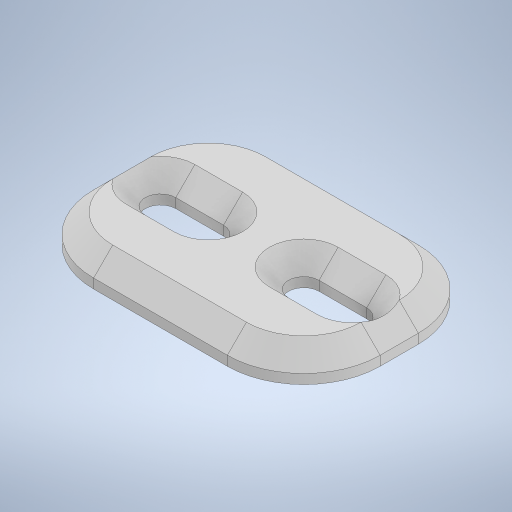
# Autodesk Inventor part: synth-straight-bracket
Saved by Autodesk Inventor 2024.1 (Build 281209000, 209)
## iProperties
Created: 2025-02-09
Part Number: synth-straight-bracket
Material: Generic
Document SubType Name: Modeling
Designer: iwheard
Density: 1 g/cm^3
Appearance: Default
Author: iwheard
Autodesk Inventor part; units mm, degrees
ref_plane "YZ Plane" through (0, 0, 0) normal (1, 0, 0) x (0, 1, 0)
ref_plane "XZ Plane" through (0, 0, 0) normal (0, 1, 0) x (-1, 0, 0)
ref_plane "XY Plane" through (0, 0, 0) normal (0, 0, 1) x (1, 0, 0)
sketch "Sketch1" plane through (0, 0, 0) normal (0, 1, 0) x (-1, 0, 0)
  line L0 (0, -20) -> (-30, -20)
  line L1 (-30, -20) -> (-30, 0)
  line L2 (-30, 0) -> (0, 0)
  line L3 (0, 0) -> (0, -20)
  dimension "d0" = 20
  dimension "d1" = 30
  constraints: 8 end point, 2 parallel, 1 coincident, 1 horizontal, 1 perpendicular
  measures "d0" distance between parallel lines of L2 L0
  measures "d1" distance between parallel lines of L3 L1
extrude "Extrusion1" add sketch "Sketch1" along normal blind 3
sketch "Sketch10" plane through (0, 3, 0) normal (0, 1, 0) x (1, 0, 0)
  circle A0 centre (5, 10) radius 1.6
  circle A1 centre (25, 10) radius 1.6
  line L0 (30, 20) -> (0, 20) projected
  line L1 (0, 0) -> (30, 0) projected
  line L2 (0, 20) -> (0, 0) projected
  line L3 (30, 0) -> (30, 20) projected
  line L4 (5, 10) -> (10, 10) construction
  line L5 (5, 8.4) -> (10, 8.4)
  line L6 (10, 11.6) -> (5, 11.6)
  arc A2 (5, 11.6) -> (5, 8.4) centre (5, 10) ccw
  arc A3 (10, 8.4) -> (10, 11.6) centre (10, 10) ccw
  line L7 (25, 10) -> (20, 10) construction
  line L8 (25, 8.4) -> (20, 8.4)
  line L9 (20, 11.6) -> (25, 11.6)
  arc A4 (25, 8.4) -> (25, 11.6) centre (25, 10) ccw
  arc A5 (20, 11.6) -> (20, 8.4) centre (20, 10) ccw
  point P0 (7.5, 10)
  point P1 (22.5, 10)
  dimension "d66" = 3.2
  dimension "d64" = 20
  dimension "d65" = 10
  dimension "d67" = 5
  dimension "d68" = 20
  dimension "d69" = 5
  dimension "d79" = 5
  dimension "d80" = 5
  constraints: 16 end point, 8 point on circle, 8 tangent, 4 centre point, 2 midpoint, 2 parallel, 1 horizontal, 1 horizontal alignment, 1 point on line, 6 other
  measures "d64" distance between parallel lines of L0 L1
  measures "d65" distance from line of L1 L4.start
  measures "d67" distance from line of L2 L4.start
  measures "d68" distance of L7.start L4.start
  measures "d69" distance from line of L3 L7.start
  measures "d79" distance of L4.end L4.start
  measures "d80" distance of L7.start L7.end
extrude "Extrusion6" cut sketch "Sketch10" against normal through all contours A0 | A0 L6 A3 L5 | A1 | A1 L8 A5 L9
fillet "Fillet5" radius 8 4 edges at (0, 1.5, 0) (0, 1.5, -20) (30, 1.5, -20) (30, 1.5, 0)
chamfer "Chamfer5" distance 2 angle 45 2 edges at (3.4, 3, -10) (26.6, 3, -10)
chamfer "Chamfer6" distance 2 angle 45 8 edges at (15, 3, 0) (27.6569, 3, -2.3431) (30, 3, -10) (27.6569, 3, -17.6569) (15, 3, -20) (2.3431, 3, -17.6569) (0, 3, -10) (2.3431, 3, -2.3431)
equation "\"d65\" = 0.5 * d64"
